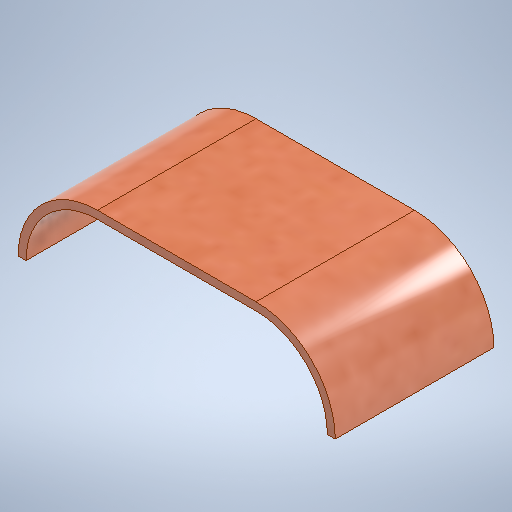
# Autodesk Inventor part: Sessao_28_03_003_001
Saved by Autodesk Inventor 2026 (Build 300175000, 175)
## iProperties
Created: 2025-04-02
Part Number: Sessao_28_03_003_001
Material: Wood (Walnut)
Document SubType Name: Modeling
Designer: Carlos Dias
Density: 0.55 g/cm^3
Appearance: Walnut - Natural Polished
Author: Carlos Dias
Autodesk Inventor part; units mm, degrees
sketch "Sketch1" plane through (0, 0, 0) normal (0, 0, 1) x (1, 0, 0)
  line L0 (-10, 10) -> (10, 10)
  arc A0 (-10, 10) -> (-20, 0) centre (-10, 0) ccw
  arc A1 (20, 0) -> (10, 10) centre (10, 0) ccw
  arc A2 (-10, 9) -> (-19, 0) centre (-10, 0) ccw
  line L1 (-10, 9) -> (10, 9)
  arc A3 (19, 0) -> (10, 9) centre (10, 0) ccw
  line L2 (-20, 0) -> (-19, 0)
  line L3 (19, 0) -> (20, 0)
  point P0 (0, 0)
  point P1 (0, 10)
  dimension "d0" = 20
  dimension "d1" = 10
  dimension "d3" = 1
  dimension "d4" = 10
  constraints: 8 end point, 8 point on circle, 4 centre point, 3 horizontal, 2 equal radius, 2 horizontal alignment, 2 tangent, 1 midpoint, 1 vertical alignment, 1 other
  measures "d0" distance of L0.start L0.end
  measures "d1" distance from line of point (0, 0) L0
  measures "d3" radial gap between concentric circles of A0 A2
  measures "d4" radius of A0
extrude "Extrusion1" add sketch "Sketch1" along normal mid plane 20
body "Solid1"
